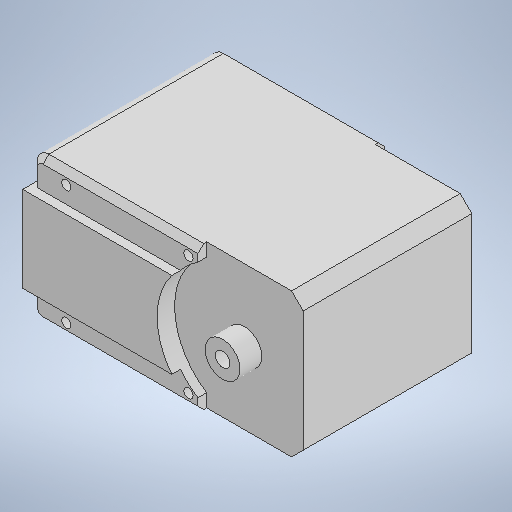
# Autodesk Inventor part: feetech-sts3215
Saved by Autodesk Inventor 2025 (Build 290162000, 162)
## iProperties
Created: 2024-07-17
Part Number: feetech-sts3215
Material: 一般
Document SubType Name: Modeling
Designer: 8326d
Density: 1 g/cm^3
Appearance: 既定
Author: 8326d
Autodesk Inventor part; units mm, degrees
ref_plane "YZ Plane" through (0, 0, 0) normal (1, 0, 0) x (0, 1, 0)
ref_plane "XZ Plane" through (0, 0, 0) normal (0, 1, 0) x (-1, 0, 0)
ref_plane "XY Plane" through (0, 0, 0) normal (0, 0, 1) x (1, 0, 0)
sketch "スケッチ1" plane through (0, 0, 0) normal (0, 0, 1) x (1, 0, 0)
  line L0 (-22.615, -12.365) -> (22.615, -12.365)
  line L1 (22.615, -12.365) -> (22.615, 12.365)
  line L2 (22.615, 12.365) -> (-22.615, 12.365)
  line L3 (-22.615, 12.365) -> (-22.615, -12.365)
  line L4 (-22.615, -12.365) -> (22.615, 12.365) construction
  line L5 (22.615, -12.365) -> (-22.615, 12.365) construction
  point P0 (0, 0)
  dimension "d0" = 45.23
  dimension "d1" = 24.73
  constraints: 12 end point, 2 midpoint, 2 parallel, 1 horizontal, 1 perpendicular
  measures "d0" distance of L2.end L1.end
  measures "d1" distance of L1.end L0.end
extrude "押し出し1" add sketch "スケッチ1" along normal mid plane 35
sketch "スケッチ2" plane through (0, 0, 17.5) normal (0, 0, 1) x (1, 0, 0)
  circle A0 centre (12.5, 0) radius 12
  line L0 (22.615, 12.365) -> (-22.615, 12.365) projected
  line L1 (6.015, 12.365) -> (6.015, -12.365)
  line L2 (-22.615, -12.365) -> (22.615, -12.365) projected
  line L3 (22.615, -12.365) -> (22.615, 12.365) projected
  point P0 (0, 0)
  point P1 (6.015, 10.0968)
  point P2 (6.015, -10.0968)
  dimension "d4" = 12.5
  dimension "d5" = 24
  dimension "d6" = 16.6
  constraints: 2 end point, 2 point on line, 1 centre point, 1 horizontal alignment, 1 vertical
  measures "d4" distance of A0.centre point (0, 0)
  measures "d5" diameter of A0
  measures "d6" distance between parallel lines of L3 L1
extrude "押し出し2" cut sketch "スケッチ2" against normal blind 3 contours L3 A0 L1 | A0 L1 L0 L3 | L3 L2 L1 A0 | L1 A0
sketch "スケッチ3" plane through (0, 0, 17.5) normal (0, 0, 1) x (1, 0, 0)
  line L0 (6.015, -12.365) -> (6.015, -10.0968) projected
  arc A0 (6.015, 10.0968) -> (6.015, -10.0968) centre (12.5, 0) ccw projected
  line L1 (6.015, 10.0968) -> (6.015, 12.365) projected
  line L2 (6.015, 12.365) -> (-22.615, 12.365) projected
  line L3 (-22.615, 12.365) -> (-22.615, -12.365) projected
  line L4 (-22.615, -12.365) -> (6.015, -12.365) projected
  line L5 (-22.615, 7.365) -> (3.026, 7.365)
  line L6 (3.026, -7.365) -> (-22.615, -7.365)
  point P0 (0, 0)
  dimension "d9" = 5
  dimension "d10" = 5
  constraints: 4 end point, 2 point on circle, 2 point on line, 1 horizontal, 1 perpendicular
  measures "d9" distance between parallel lines of L2 L5
  measures "d10" distance between parallel lines of L4 L6
extrude "押し出し3" cut sketch "スケッチ3" against normal blind 1.5 contours L4 L3 L6 A0 L0 | L5 L3 L2 L1 A0
sketch "スケッチ4" plane through (0, 0, 14.5) normal (0, 0, 1) x (1, 0, 0)
  arc A0 (6.015, 10.0968) -> (3.026, 7.365) centre (12.5, 0) ccw projected
  circle A1 centre (12.5, 0) radius 3
  point P0 (0, 0)
  dimension "d13" = 6
  constraints: 1 centre point, 1 coincident
  measures "d13" diameter of A1
extrude "押し出し4" add sketch "スケッチ4" along normal blind 3.75
sketch "スケッチ9" plane through (12.5, 0, 18.25) normal (0, 0, 1) x (1, 0, 0)
  circle A0 centre (0, 0) radius 3 projected
  point P0 (-12.5, 0)
hole "穴3" at (12.5, 0, 18.25) direction (0, 0, -1) diameter 2.5 depth 8 tip angle 118
fillet "フィレット2" radius 2 2 edges at (-22.615, 12.365, -0.75) (-22.615, -12.365, -0.75)
chamfer "面取り1" distance 1 angle 45 4 edges at (-7.3, 12.365, 16) (-22.615, 8.865, 16) (-22.615, -8.865, 16) (-7.3, -12.365, 16)
mirror "ミラー1" about plane through (0, 0, 0) normal (0, 0, 1) of "押し出し2", "押し出し3", "押し出し4", "面取り1", "穴3"
chamfer "面取り2" distance 2 angle 45 2 edges at (22.615, 12.365, 0) (22.615, -12.365, 0)
sketch "スケッチ5" plane through (0, 0, 16) normal (0, 0, 1) x (1, 0, 0)
  line L0 (-16.615, -10.25) -> (4.385, -10.25) construction
  line L1 (4.385, -10.25) -> (4.385, 10.25) construction
  line L2 (4.385, 10.25) -> (-16.615, 10.25) construction
  line L3 (-16.615, 10.25) -> (-16.615, -10.25) construction
  line L4 (-16.615, -10.25) -> (4.385, 10.25) construction
  line L5 (4.385, -10.25) -> (-16.615, 10.25) construction
  line L6 (-22.615, 7.365) -> (-22.615, 12.365) construction
  point P0 (0, 0)
  point P1 (-6.115, 0)
  dimension "d16" = 21
  dimension "d17" = 20.5
  dimension "d18" = 6
  constraints: 12 end point, 2 midpoint, 2 parallel, 1 horizontal, 1 horizontal alignment, 1 perpendicular
  measures "d16" distance of L2.end L1.end
  measures "d17" distance of L1.end L0.end
  measures "d18" distance between parallel lines of L6 L3
hole "穴1" at (-16.615, 10.25, 16) at (-16.615, -10.25, 16) at (4.385, -10.25, 16) at (4.385, 10.25, 16) direction (0, 0, -1) diameter 1.6 depth 8 tip angle 118
sketch "スケッチ6" plane through (6.015, 11.365, -16) normal (0, 0, -1) x (-1, 0, 0)
  circle A0 centre (1.63, -1.115) radius 0.8 projected
  circle A1 centre (1.63, -1.115) radius 0.8 projected
  circle A2 centre (1.63, -21.615) radius 0.8 projected
  circle A3 centre (1.63, -21.615) radius 0.8 projected
  line L0 (1.63, -1.115) -> (26.63, -1.115)
  line L1 (26.63, -1.115) -> (26.63, -21.615)
  line L2 (26.63, -21.615) -> (1.63, -21.615)
  line L3 (1.63, -21.615) -> (1.63, -1.115)
  point P0 (6.015, -11.365)
  dimension "d34" = 25
  constraints: 8 end point, 2 parallel, 1 coincident, 1 horizontal, 1 perpendicular
  measures "d34" distance of L0.start L0.end
hole "穴2" at (4.385, 10.25, -16) at (-20.615, 10.25, -16) at (-20.615, -10.25, -16) at (4.385, -10.25, -16) direction (0, 0, 1) diameter 1.6 depth 8 tip angle 118
sketch "スケッチ7" plane through (0, 0, -17.5) normal (0, 0, -1) x (-1, 0, 0)
  circle A0 centre (-12.5, 0) radius 3 projected
  line L0 (-0.4, -10) -> (5.6, -10)
  line L1 (5.6, -10) -> (5.6, 10)
  line L2 (5.6, 10) -> (-0.4, 10)
  line L3 (-0.4, 10) -> (-0.4, -10)
  line L4 (-0.4, -10) -> (5.6, 10) construction
  line L5 (5.6, -10) -> (-0.4, 10) construction
  arc A1 (-3.026, 7.365) -> (-6.015, 10.0968) centre (-12.5, 0) ccw projected
  line L6 (-2.4, 6.48) -> (-0.4, 6.48)
  line L7 (-0.4, 6.48) -> (-0.4, -6.48)
  line L8 (-0.4, -6.48) -> (-2.4, -6.48)
  line L9 (-2.4, -6.48) -> (-2.4, 6.48)
  arc A2 (-3.026, -7.365) -> (-3.026, 7.365) centre (-12.5, 0) ccw projected
  point P0 (0, 0)
  point P1 (2.6, 0)
  point P2 (-2.4, 0)
  point P3 (-0.5, 0)
  point P4 (-0.4, 6.48)
  dimension "d42" = 6
  dimension "d43" = 20
  dimension "d44" = 12.96
  dimension "d45" = 2
  constraints: 20 end point, 4 parallel, 3 midpoint, 2 horizontal, 2 horizontal alignment, 2 perpendicular, 2 point on circle, 1 point on line
  measures "d42" distance of L2.end L1.end
  measures "d43" distance of L1.end L0.end
  measures "d44" distance of L8.end L6.start
  measures "d45" distance of L6.start L6.end
extrude "押し出し5" cut sketch "スケッチ7" against normal up to surface (3 mm away) contours L3 L2 L1 L0 | L8 A2 L6 L3 | L9 A2
sketch "スケッチ8" plane through (0, 0, -17.5) normal (0, 0, -1) x (-1, 0, 0)
  line L0 (-2.4, 6.48) -> (-0.4, 6.48) projected
  line L1 (-0.4, 6.48) -> (-0.4, 7.365) projected
  line L2 (-0.4, 7.365) -> (-3.026, 7.365) projected
  arc A0 (-2.4, 6.48) -> (-3.026, 7.365) centre (-12.5, 0) ccw projected
  line L3 (-0.4, -6.48) -> (-2.4, -6.48) projected
  arc A1 (-3.026, -7.365) -> (-2.4, -6.48) centre (-12.5, 0) ccw projected
  line L4 (-3.026, -7.365) -> (-0.4, -7.365) projected
  line L5 (-0.4, -7.365) -> (-0.4, -6.48) projected
  point P0 (0, 0)
extrude "押し出し6" cut sketch "スケッチ8" against normal up to surface (1.5 mm away)
chamfer "面取り3" distance 1.5 angle 45 1 edges at (-5.6, 0, -17.5)
equation "\"d10\" = d9"
